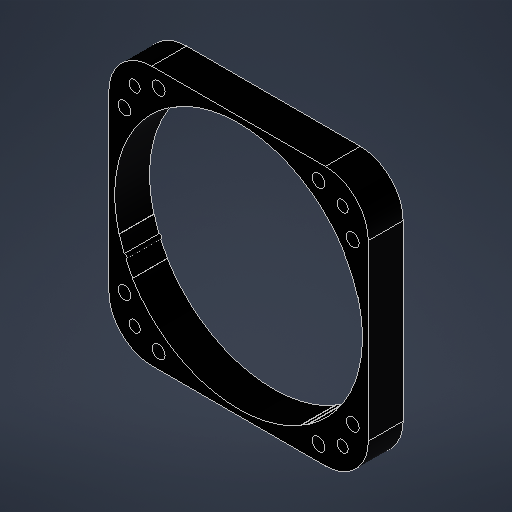
# Autodesk Inventor part: stator_center_00_p
Saved by Autodesk Inventor 2026.1 (Build 301233000, 233)
## iProperties
Created: 2026-04-12
Part Number: stator_center_00_p
Material: PC/ABS Plastic
Document SubType Name: Modeling
Designer: aaron
Density: 1.1 g/cm^3
Appearance: Smooth - White
Author: aaron
Autodesk Inventor part; units mm, degrees
ref_plane "YZ Plane" through (0, 0, 0) normal (1, 0, 0) x (0, 1, 0)
ref_plane "XZ Plane" through (0, 0, 0) normal (0, 1, 0) x (-1, 0, 0)
ref_plane "XY Plane" through (0, 0, 0) normal (0, 0, 1) x (1, 0, 0)
sketch "Sketch1" plane through (0, 0, 0) normal (0, 0, 1) x (1, 0, 0)
  circle A0 centre (0, 0) radius 57.5
  circle A1 centre (0, 0) radius 60.5
  line L0 (-40.5, 60.5) -> (40.5, 60.5)
  line L1 (60.5, 40.5) -> (60.5, -40.5)
  line L2 (40.5, -60.5) -> (-40.5, -60.5)
  line L3 (-60.5, -40.5) -> (-60.5, 40.5)
  arc A2 (-40.5, 60.5) -> (-60.5, 40.5) centre (-40.5, 40.5) ccw
  arc A3 (60.5, 40.5) -> (40.5, 60.5) centre (40.5, 40.5) ccw
  arc A4 (40.5, -60.5) -> (60.5, -40.5) centre (40.5, -40.5) ccw
  arc A5 (-60.5, -40.5) -> (-40.5, -60.5) centre (-40.5, -40.5) ccw
  dimension "d0" = 115
  dimension "d1" = 121
  dimension "d2" = 20
  constraints: 12 tangent, 8 end point, 8 point on circle, 6 centre point, 3 equal radius, 2 coincident, 2 parallel, 1 horizontal, 1 perpendicular
  measures "d0" diameter of A0
  measures "d1" diameter of A1
  measures "d2" radius of A2
extrude "Extrusion1" add sketch "Sketch1" along normal blind 16.25
sketch "Sketch3" plane through (0, 0, 16.25) normal (0, 0, 1) x (1, 0, 0)
  circle A0 centre (-48.5, -48.5) radius 2.65 projected
  circle A1 centre (-53.2449, -37.2825) radius 2.15 projected
  circle A2 centre (-37.2825, -53.2449) radius 2.15 projected
  circle A3 centre (37.2825, -53.2449) radius 2.15 projected
  circle A4 centre (48.5, -48.5) radius 2.65 projected
  circle A5 centre (53.2449, -37.2825) radius 2.15 projected
  circle A6 centre (53.2449, 37.2825) radius 2.15 projected
  circle A7 centre (48.5, 48.5) radius 2.65 projected
  circle A8 centre (37.2825, 53.2449) radius 2.15 projected
  circle A9 centre (-37.2825, 53.2449) radius 2.15 projected
  circle A10 centre (-48.5, 48.5) radius 2.65 projected
  circle A11 centre (-53.2449, 37.2825) radius 2.15 projected
  point P0 (0, 0)
extrude "Extrusion3" cut sketch "Sketch3" against normal through all
sketch "Sketch4" plane through (0, 0, 16.25) normal (0, 0, 1) x (1, 0, 0)
  circle A0 centre (-37.2825, -53.2449) radius 2.15 projected
  circle A1 centre (-37.2825, -53.2449) radius 3
  circle A2 centre (-53.2449, -37.2825) radius 2.15 projected
  circle A3 centre (-53.2449, -37.2825) radius 3
  circle A4 centre (-53.2449, 37.2825) radius 2.15 projected
  circle A5 centre (-53.2449, 37.2825) radius 3
  circle A6 centre (-37.2825, 53.2449) radius 2.15 projected
  circle A7 centre (-37.2825, 53.2449) radius 3
  circle A8 centre (37.2825, 53.2449) radius 2.15 projected
  circle A9 centre (37.2825, 53.2449) radius 3
  circle A10 centre (53.2449, 37.2825) radius 2.15 projected
  circle A11 centre (53.2449, 37.2825) radius 3
  circle A12 centre (53.2449, -37.2825) radius 2.15 projected
  circle A13 centre (53.2449, -37.2825) radius 3
  circle A14 centre (37.2825, -53.2449) radius 2.15 projected
  circle A15 centre (37.2825, -53.2449) radius 3
  point P0 (0, 0)
  point P1 (48.5, -48.5)
  dimension "d28" = 6
  dimension "d29" = 6
  dimension "d30" = 6
  dimension "d31" = 6
  dimension "d32" = 6
  dimension "d33" = 6
  dimension "d34" = 6
  dimension "d36" = 6
  constraints: 8 centre point, 8 coincident
  measures "d28" diameter of A1
  measures "d29" diameter of A3
  measures "d30" diameter of A5
  measures "d31" diameter of A7
  measures "d32" diameter of A9
  measures "d33" diameter of A11
  measures "d34" diameter of A13
  measures "d36" diameter of A15
extrude "Extrusion4" cut sketch "Sketch4" against normal through all contours A0 | A1 | A2 | A3 | A4 | A5 | A6 | A7 | A8 | A9 | A10 | A11 | A12 | A13 | A14 | A15
sketch "Sketch5" plane through (0, 0, 16.25) normal (0, 0, 1) x (1, 0, 0)
  arc A0 (-51.9873, -22.1262) -> (-53.291, -21.5943) centre (-52.9074, -22.5178) ccw
  arc A1 (-52.5078, -23.4345) -> (-51.9873, -22.1262) centre (-52.9074, -22.5178) ccw
  circle A2 centre (0, 0) radius 57.55
  circle A3 centre (-52.9074, -22.5178) radius 0.95
  circle A4 centre (0, 0) radius 57.75
  line L0 (55.7822, 14.9468) -> (-70.3053, -18.8382)
  line L1 (40.5, 60.5) -> (-40.5, 60.5) projected
  line L2 (49.5014, 29.7434) -> (-78.6926, -47.2833)
  line L3 (32.5757, -47.6853) -> (-33.549, 49.11)
  line L4 (29.1077, -49.8779) -> (-30.5513, 52.3515)
  point P0 (-55.7822, -14.9468)
  point P1 (-55.589, -14.895)
  point P2 (-53.3179, -21.6611)
  point P3 (-52.5746, -23.4076)
  point P4 (-49.33, -29.6404)
  point P5 (-49.5014, -29.7434)
  point P6 (29.0069, -49.7051)
  point P7 (32.4629, -47.5201)
  point P8 (-29.1077, 49.8779)
  point P9 (-29.0069, 49.7051)
  point P10 (-32.4629, 47.5201)
  point P11 (-32.5757, 47.6853)
  dimension "d39" = 115.1
  dimension "d40" = 115.5
  dimension "d41" = 15
  dimension "d42" = 16
  constraints: 8 end point, 8 point on circle, 5 centre point, 4 point on line, 3 coincident, 7 other
  measures "d39" diameter of A2
  measures "d40" diameter of A4
  measures "d41" angle of L1 L0
  measures "d42" angle of L2 L0
extrude "Extrusion5" cut sketch "Sketch5" against normal through all contours A2 L3 L0 | A2 L0 A4 L3 | A2 L4 L3 | L2 L4 A2 | A2 L4 A4 L2 | L2 A2 A3 L0 | L4 A2 L2 | L0 A2 L3 | L3 A2 L4 | L4 A4 L2 A2 | L0 A4 L3 A2
sketch "Sketch6" plane through (0, 0, 16.25) normal (0, 0, 1) x (1, 0, 0)
  arc A0 (-52.5078, -23.4345) -> (-51.9873, -22.1262) centre (-52.9074, -22.5178) ccw
  arc A1 (-51.9873, -22.1262) -> (-53.291, -21.5943) centre (-52.9074, -22.5178) ccw
  arc A2 (-53.2722, -21.6407) -> (-52.5282, -23.3888) centre (0, 0) ccw projected
  circle A3 centre (-52.9074, -22.5178) radius 0.95
  point P0 (-52.5282, -23.3888)
  constraints: 4 point on circle, 2 centre point, 1 coincident, 10 other
extrude "Extrusion6" add sketch "Sketch6" against normal up to surface (16.25 mm away) contours A3 A2 picked at (-52.6277, -22.3682)
equation "\"d28\" = d31"
equation "\"d29\" = d31"
equation "\"d30\" = d31"
equation "\"d32\" = d31"
equation "\"d33\" = d31"
equation "\"d34\" = d31"
equation "\"d36\" = d31"
body "Solid1"
